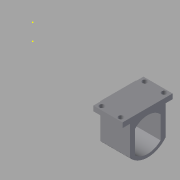
# Autodesk Inventor part: smallpart
Saved by Autodesk Inventor 2015 (Build 190159000, 159)
## iProperties
Created: 2015-11-09
Part Number: smallpart
Material: Generic
Document SubType Name: Modeling
Designer: Ross
Density: 1 g/cm^3
Appearance: Default
Author: Ross
Autodesk Inventor part; units mm, degrees
ref_plane "YZ Plane" through (0, 0, 0) normal (1, 0, 0) x (0, 1, 0)
ref_plane "XZ Plane" through (0, 0, 0) normal (0, 1, 0) x (-1, 0, 0)
ref_plane "XY Plane" through (0, 0, 0) normal (0, 0, 1) x (1, 0, 0)
sketch "Sketch1" plane through (0, 0, 0) normal (0, 1, 0) x (-1, 0, 0)
  line L0 (70, 0) -> (70, -70)
  line L1 (70, -70) -> (0, -70)
  line L2 (-70, 0) -> (-70, 70)
  line L3 (-70, 70) -> (0, 70)
  line L4 (0, 70) -> (70, 70)
  line L5 (70, 70) -> (70, 0)
  line L6 (0, -70) -> (-70, -70)
  line L7 (-70, -70) -> (-70, 0)
  point P0 (0, 0)
  constraints: 16 end point, 4 perpendicular, 2 point on line, 1 vertical
extrude "Extrusion1" add sketch "Sketch1" along normal blind 3
fillet "Fillet1" radius 5 3 edges at (70, 1.5, 70) (70, 1.5, -70) (-70, 1.5, 70)
fillet "Fillet2" radius 5 1 edges at (-70, 1.5, -70)
ref_plane "Work Plane1" through (65, 0, 65) normal (1, 0, 0) x (0, 0, -1)
sketch "Sketch6" plane through (70, 0, 65) normal (1, 0, 0) x (0, 0, -1)
  line L0 (65, 0) -> (57.2, 0)
  line L1 (130, 0) -> (0, 0) projected
  line L2 (65, 0) -> (72.8, 0)
  line L3 (57.2, 0) -> (57.2, -18)
  line L4 (72.8, 0) -> (72.8, -18)
  line L5 (65, 0) -> (65, -10)
  arc A0 (57.2, -18) -> (72.8, -18) centre (65, -10.2437) ccw
  line L6 (57.2, 0) -> (54.2, 0)
  line L7 (54.2, 0) -> (54.2, -18)
  line L8 (72.8, 0) -> (75.8, 0)
  line L9 (75.8, 0) -> (75.8, -18)
  arc A1 (54.2, -18) -> (75.8, -18) centre (65, -9.0916) ccw
  dimension "d17" = 18
  dimension "d21" = 3
  dimension "d22" = 3
  constraints: 18 end point, 4 point on circle, 4 point on line, 3 perpendicular, 2 centre point, 2 vertical
  measures "d17" distance of L0.end L3.end
  measures "d21" distance of L0.end L6.end
  measures "d22" distance of L2.end L8.end
extrude "Extrusion3" add sketch "Sketch6" against normal blind 18 contours L3 A0 L4 L1 L9 A1 L7
pattern_circular "Circular Pattern1" count 4 over 360 about axis through (0, -10, 0) along (0, 1, 0) of "Extrusion3"
sketch "Sketch8" plane through (0, 3, 0) normal (0, 1, 0) x (1, 0, 0)
  circle A0 centre (58.4636, -19.348) radius 2.5
  point P0 (0, 0)
  dimension "d35" = 5
  constraints: 1 centre point
  measures "d35" diameter of A0
extrude "Extrusion5" cut sketch "Sketch8" against normal blind 3
sketch "Sketch9" plane through (0, 3, 0) normal (0, 1, 0) x (1, 0, 0)
  circle A0 centre (-60.6489, 18.9578) radius 2.5
  point P0 (0, 0)
  dimension "d39" = 5
  constraints: 1 centre point
  measures "d39" diameter of A0
extrude "Extrusion6" cut sketch "Sketch9" against normal blind 3
sketch "Sketch10" plane through (0, 3, 0) normal (0, 1, 0) x (1, 0, 0)
  line L0 (70, -65) -> (70, 65) projected
  line L1 (70, 15.1257) -> (39.2687, 15.1257)
  line L2 (39.2687, 15.1257) -> (39.2687, -15.3197)
  line L3 (39.2687, -15.3197) -> (70, -15.3197)
  line L4 (70, -15.3197) -> (70, 15.1257)
  point P0 (0, 0)
  constraints: 8 end point, 2 parallel, 1 horizontal, 1 perpendicular, 1 point on line
extrude "Extrusion7" add sketch "Sketch10" along normal blind 10
sketch "Sketch11" plane through (0, 3, 0) normal (0, 1, 0) x (1, 0, 0)
  point P0 (0, 0)
sketch "Sketch12" plane through (0, 3, 0) normal (0, 1, 0) x (1, 0, 0)
  line L0 (39.2687, -15.3197) -> (39.2687, -70)
  line L1 (10.8, -70) -> (65, -70) projected
  line L2 (39.2687, -15.3197) -> (39.2687, 15.1257) projected
  line L3 (39.2687, -70) -> (-73.9803, -70)
  line L4 (-73.9803, -70) -> (-73.9803, 75.2408)
  line L5 (-73.9803, 75.2408) -> (39.2687, 75.2408)
  line L6 (39.2687, 75.2408) -> (39.2687, -70)
  point P0 (0, 0)
  constraints: 10 end point, 2 parallel, 1 collinear, 1 horizontal, 1 perpendicular, 1 point on line
extrude "Extrusion8" cut sketch "Sketch12" against normal blind 100
sketch "Sketch13" plane through (0, 3, 0) normal (0, 1, 0) x (1, 0, 0)
  line L0 (39.2687, -15.3197) -> (74.5621, -15.3197)
  line L1 (74.5621, -15.3197) -> (74.5621, -76.2104)
  line L2 (74.5621, -76.2104) -> (39.2687, -76.2104)
  line L3 (39.2687, -76.2104) -> (39.2687, -15.3197)
  point P0 (0, 0)
  constraints: 8 end point, 2 parallel, 1 horizontal, 1 perpendicular
extrude "Extrusion9" cut sketch "Sketch13" against normal blind 100
sketch "Sketch14" plane through (0, 3, 0) normal (0, 1, 0) x (1, 0, 0)
  line L0 (39.2687, 15.1257) -> (72.3919, 15.1257)
  line L1 (72.3919, 15.1257) -> (72.3919, 74.5163)
  line L2 (72.3919, 74.5163) -> (39.2687, 74.5163)
  line L3 (39.2687, 74.5163) -> (39.2687, 15.1257)
  point P0 (0, 0)
  constraints: 8 end point, 2 parallel, 1 horizontal, 1 perpendicular
extrude "Extrusion10" cut sketch "Sketch14" against normal blind 100
sketch "Sketch15" plane through (0, 13, 0) normal (0, 1, 0) x (1, 0, 0)
  point P0 (0, 0)
sketch "Sketch17" plane through (70, -18, 10.8) normal (1, 0, 0) x (0, 0, -1)
  line L0 (-4.5197, 18) -> (-4.5197, 21)
  line L1 (-4.5197, 18) -> (-4.5197, 31) projected
  line L2 (-4.5197, 21) -> (25.9257, 21)
  line L3 (25.9257, 31) -> (25.9257, 18) projected
  line L4 (25.9257, 21) -> (-4.5197, 21)
  line L5 (-4.5197, 21) -> (-4.5197, 31)
  line L6 (-4.5197, 31) -> (25.9257, 31)
  line L7 (25.9257, 31) -> (25.9257, 21)
  point P0 (10.8, 18)
  dimension "d50" = 3
  constraints: 12 end point, 2 parallel, 2 perpendicular, 2 point on line, 1 horizontal
  measures "d50" distance of L0.start L0.end
extrude "Extrusion11" cut sketch "Sketch17" against normal blind 100
sketch "Sketch18" plane through (39.2687, 0, -15.1257) normal (-1, 0, 0) x (0, 0, 1)
  line L0 (0, 3) -> (30.4454, 3)
  line L1 (30.4454, 3) -> (30.4454, 0)
  line L2 (30.4454, 0) -> (0, 0)
  line L3 (0, 0) -> (0, 3)
  point P0 (15.1257, 0)
  constraints: 8 end point, 2 parallel, 1 horizontal, 1 perpendicular
extrude "Extrusion12" cut sketch "Sketch18" against normal blind 13
sketch "Sketch20" plane through (52, 0, 65) normal (-1, 0, 0) x (0, 0, 1)
  line L0 (-72.8, -18) -> (-72.8, 0) projected
  line L1 (-72.8, -9) -> (-57.2, -9)
  line L2 (-57.2, -18) -> (-57.2, 0) projected
  line L3 (-72.8, -18) -> (-72.8, -4)
  arc A0 (-72.8, -18) -> (-57.2, -18) centre (-65, -10.2437) ccw projected
  line L4 (-65, -21.2437) -> (-72.8, -21.2437)
  line L5 (-72.8, -4) -> (-72.8, -0.8)
  line L6 (-65, -21.2437) -> (-65, -3.2437)
  line L7 (-65, -21.2437) -> (-65, -11.2437)
  line L8 (-65, -11.2437) -> (-65, -1.2437)
  line L9 (-65, -1.2437) -> (-65, -0.8)
  arc A1 (-65, -0.8) -> (-72.6527, -4.1368) centre (-65, -11.2437) ccw
  arc A2 (-57.2, -4.2988) -> (-65, -0.8) centre (-65, -11.2437) ccw
  arc A3 (-72.6527, -4.1368) -> (-72.8, -4.2988) centre (-65, -11.2437) ccw
  arc A4 (-57.2, -4.2988) -> (-57.2, -4.2988) centre (-65, -11.2437) ccw
  line L10 (-72.8, -4.2988) -> (-72.8, 0)
  line L11 (-57.2, 0) -> (-57.2, -4.2988)
  line L12 (-57.2, 0) -> (-72.8, 0) projected
  line L13 (-57.2, -4.2988) -> (-57.2, 0)
  line L14 (-72.8, -4.2988) -> (-72.8, 0)
  line L15 (-72.8, 0) -> (-57.2, 0)
  point P0 (-65, 0)
  dimension "d55" = 14
  dimension "d56" = 3.2
  dimension "d57" = 18
  dimension "d58" = 10
  dimension "d59" = 10
  constraints: 26 end point, 9 point on circle, 4 centre point, 4 coincident, 4 point on line, 3 collinear, 2 midpoint, 2 vertical, 1 horizontal, 1 perpendicular, 1 tangent
  measures "d55" distance of L0.start L3.end
  measures "d56" distance of L3.end L5.end
  measures "d57" distance of L4.start L6.end
  measures "d58" distance of L4.start L7.end
  measures "d59" distance of L7.end L8.end
extrude "Extrusion13" add sketch "Sketch20" against normal blind 18 contours L0 L12 L2 A2 A1 A3
sketch "Sketch22" plane through (52.2687, 0, 10.8) normal (0, 1, 0) x (1, 0, 0)
  line L0 (-0.2687, 21.6) -> (0, 21.6)
  line L1 (0, 21.6) -> (0, 0)
  line L2 (0, 0) -> (-0.2687, 0)
  line L3 (-0.2687, 0) -> (-0.2687, 21.6)
  point P0 (-52.2687, 10.8)
  constraints: 8 end point, 2 parallel, 1 horizontal, 1 perpendicular
extrude "Extrusion14" add sketch "Sketch22" along normal blind 3
sketch "Sketch23" plane through (70, 3, 15.3197) normal (0, 1, 0) x (1, 0, 0)
  line L0 (-17.7313, 30.4454) -> (-17.7313, 26.1197)
  line L1 (0, 26.1197) -> (-17.7313, 26.1197) projected
  line L2 (-17.7313, 28.2825) -> (0, 28.2825)
  line L3 (0, 30.4454) -> (0, 0) projected
  circle A0 centre (-14.6963, 28.2825) radius 1.5
  line L4 (0, 28.2825) -> (-3, 28.2825)
  circle A1 centre (-3, 28.2825) radius 1.5
  line L5 (0, 30.4454) -> (0, 0)
  line L6 (0, 23.1197) -> (-18, 23.1197) projected
  line L7 (0, 15.2227) -> (-18, 15.3197)
  line L8 (-18, 26.1197) -> (-18, 4.5197) projected
  circle A2 centre (-14.8362, 2.3219) radius 1.5
  circle A3 centre (-3.1405, 2.1959) radius 1.5
  point P0 (-70, 15.3197)
  dimension "d64" = 3
  dimension "d65" = 3
  dimension "d66" = 3
  constraints: 10 end point, 4 centre point, 3 midpoint, 3 point on line, 2 perpendicular, 2 symmetric about line, 1 coincident, 1 horizontal, 2 other
  measures "d64" diameter of A0
  measures "d65" distance of L2.end L4.end
  measures "d66" diameter of A1
extrude "Extrusion15" cut sketch "Sketch23" against normal blind 4 contours A0 L2 | L2 A0 | A1 L2 | L2 A1 | A2 | A3
body "Solid1"
